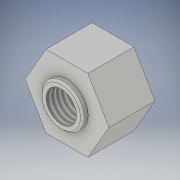
# Autodesk Inventor part: Нагаечник
Saved by Autodesk Inventor 2017 (Build 210142000, 142)
## iProperties
Part Number: Нагаечник
Material: Типовые
Document SubType Name: Modeling
Designer: Daemon
Density: 1 g/cm^3
Appearance: По умолчанию
Author: Daemon
Autodesk Inventor part; units mm, degrees
ref_plane "YZ Plane" through (0, 0, 0) normal (1, 0, 0) x (0, 1, 0)
ref_plane "XZ Plane" through (0, 0, 0) normal (0, 1, 0) x (-1, 0, 0)
sketch "Эскиз1" plane through (0, 0, 0) normal (0, 0, 1) x (1, 0, 0)
  circle A0 centre (0, 0) radius 4
  line L0 (10.9362, 0) -> (5.4681, 9.471)
  line L1 (-5.4681, 9.471) -> (5.4681, 9.471)
  line L2 (-10.9362, 0) -> (-5.4681, 9.471)
  line L3 (-5.4681, -9.471) -> (5.4681, -9.471)
  line L4 (-5.4681, -9.471) -> (-10.9362, 0)
  line L5 (10.9362, 0) -> (5.4681, -9.471)
  line L6 (0, 0) -> (10.9362, 0)
  dimension "d45" = 8
  dimension "d52" = 120
  dimension "d53" = 120
  dimension "d54" = 10.9362
  dimension "d55" = 9.471
  constraints: 14 end point, 3 equal length, 3 parallel, 2 horizontal, 1 centre point, 1 coincident
  measures "d45" diameter of A0
  measures "d52" angle of L0 L1
  measures "d53" angle of L3 L5
  measures "d54" distance of L3.start L3.end
  measures "d55" distance from line of point (0, 0) L5
extrude "Выдавливание1" add sketch "Эскиз1" along normal blind 12
sketch "Эскиз3" plane through (0, 0, 12) normal (0, 0, 1) x (1, 0, 0)
  circle A0 centre (0, 0) radius 4
  circle A1 centre (0, 0) radius 5.5
  dimension "d56" = 8
  dimension "d57" = 11
  constraints: 2 centre point, 2 coincident
  measures "d56" diameter of A0
  measures "d57" diameter of A1
extrude "Выдавливание3" add sketch "Эскиз3" along normal blind 1.5
chamfer "Фаска2" distance 0.5 angle 45 1 edges at (-5.5, 0, 13.5)
ref_plane "РабПлоскость1" through (0, 0, 6) normal (0, 0, 1) x (1, 0, 0)
mirror "Зеркальное отражение1" about plane through (0, 0, 6) normal (0, 0, 1) of "Выдавливание3"
chamfer "Фаска3" distance 0.5 angle 45 1 edges at (-5.5, 0, -1.5)
thread "Резьба1" size "M8x1.25" class "6H" standard "ANSI Metric M Profile" full length
